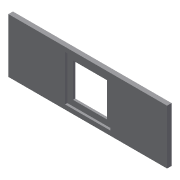
# Autodesk Inventor part: cellSTORM_coverslip_slide_adapter
Saved by Autodesk Inventor 2019 (Build 230136000, 136)
## iProperties
Created: 2019-12-13
Part Number: cellSTORM_coverslip_slide_adapter
Material: Generic
Document SubType Name: Modeling
Designer: diederichbenedict
Density: 1 g/cm^3
Appearance: Default
Author: diederichbenedict
Autodesk Inventor part; units mm, degrees
ref_plane "YZ Plane" through (0, 0, 0) normal (1, 0, 0) x (0, 1, 0)
ref_plane "XZ Plane" through (0, 0, 0) normal (0, 1, 0) x (-1, 0, 0)
ref_plane "XY Plane" through (0, 0, 0) normal (0, 0, 1) x (1, 0, 0)
sketch "Sketch1" plane through (0, 0, 0) normal (0, 0, 1) x (1, 0, 0)
  line L0 (0, 0) -> (70, 0)
  line L1 (70, 0) -> (70, 24)
  line L2 (70, 24) -> (0, 24)
  line L3 (0, 24) -> (0, 0)
  line L4 (27.5, 4.5) -> (42.5, 4.5)
  line L5 (42.5, 4.5) -> (42.5, 19.5)
  line L6 (42.5, 19.5) -> (27.5, 19.5)
  line L7 (27.5, 19.5) -> (27.5, 4.5)
  line L8 (27.5, 4.5) -> (42.5, 19.5) construction
  line L9 (42.5, 4.5) -> (27.5, 19.5) construction
  point P0 (35, 12)
  dimension "d0" = 70
  dimension "d1" = 24
  dimension "d2" = 15
  dimension "d3" = 15
  constraints: 20 end point, 4 parallel, 2 horizontal, 2 midpoint, 2 perpendicular
  measures "d0" distance of L2.end L1.end
  measures "d1" distance of L1.end L0.end
  measures "d2" distance of L6.end L5.end
  measures "d3" distance of L5.end L4.end
extrude "Extrusion1" add sketch "Sketch1" along normal blind 1
sketch "Sketch2" plane through (0, 0, 1) normal (0, 0, 1) x (1, 0, 0)
  line L0 (27.5, 4.5) -> (27.5, 19.5) projected
  line L1 (27.5, 19.5) -> (42.5, 19.5) projected
  line L2 (42.5, 19.5) -> (42.5, 4.5) projected
  line L3 (42.5, 4.5) -> (27.5, 4.5) projected
  line L4 (0, 0) -> (70, 0) projected
  line L5 (70, 0) -> (70, 24) projected
  line L6 (70, 24) -> (0, 24) projected
  line L7 (0, 24) -> (0, 0) projected
  line L8 (45, 2) -> (25, 2)
  line L9 (25, 2) -> (25, 22)
  line L10 (25, 22) -> (45, 22)
  line L11 (45, 22) -> (45, 2)
  line L12 (45, 2) -> (25, 22) construction
  line L13 (25, 2) -> (45, 22) construction
  point P0 (35, 12)
  dimension "d6" = 20
  dimension "d7" = 20
  constraints: 12 end point, 2 midpoint, 2 parallel, 1 horizontal, 1 perpendicular
  measures "d6" distance of L9.end L10.end
  measures "d7" distance of L8.end L9.end
extrude "Extrusion2" add sketch "Sketch2" along normal blind 1 contours L7 L6 L5 L4
body "Solid1"
